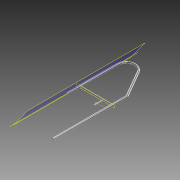
# Autodesk Inventor part: Geländer lang
Saved by Autodesk Inventor 2019 (Build 230136000, 136)
## iProperties
Created: 2017-04-11
Part Number: Geländer lang
Material: Allgemein
Document SubType Name: Modeling
Designer: Seelenernter
Density: 1 g/cm^3
Appearance: Chrom - poliert
Author: Seelenernter
Autodesk Inventor part; units mm, degrees
ref_plane "YZ Plane" through (0, 0, 0) normal (1, 0, 0) x (0, 1, 0)
ref_plane "XY Plane" through (0, 0, 0) normal (0, 0, 1) x (1, 0, 0)
sketch "Skizze1" plane through (0, 0, 0) normal (0, 1, 0) x (-1, 0, 0)
  circle A0 centre (0, 0) radius 20
  dimension "d0" = 40
  constraints: 1 centre point, 1 coincident
  measures "d0" diameter of A0
sketch "Skizze2" plane through (0, 0, 0) normal (0, 0, 1) x (1, 0, 0)
  line L0 (0, 0) -> (0, 770)
  line L1 (180, 950) -> (183.4788, 950)
  line L2 (356.6838, 850) -> (680, 290)
  line L3 (680, 290) -> (680, -1250)
  arc A0 (180, 950) -> (0, 770) centre (180, 770) ccw
  arc A1 (356.6838, 850) -> (183.4788, 950) centre (183.4788, 750) ccw
  point P0 (0, 950)
  dimension "d1" = 950
  dimension "d4" = 290
  dimension "d8" = 2200
  dimension "d9" = 30
  dimension "d10" = 680
  dimension "d11" = 180
  dimension "d12" = 200
  constraints: 8 end point, 4 point on circle, 4 tangent, 2 centre point, 2 point on line, 2 vertical, 1 perpendicular
  measures "d1" distance of L0.start point (0, 950)
  measures "d4" vertical distance of L2.end L0.start
  measures "d8" distance from line of L3.end L1
  measures "d9" angle of L2 L3
  measures "d10" distance between parallel lines of L0 L3
  measures "d11" radius of A0
  measures "d12" radius of A1
sweep "Sweeping1" add profiles "Skizze1" path "Skizze2"
sketch "Skizze3" plane through (0, 0, 0) normal (1, 0, 0) x (0, 1, 0)
  circle A0 centre (-20, 0) radius 15
  line L0 (0, 20) -> (0, -20) projected
  point P0 (0, 0)
  point P1 (0, 0)
  dimension "d16" = 30
  dimension "d27" = 20
  constraints: 1 centre point, 1 horizontal alignment, 1 midpoint
  measures "d16" diameter of A0
  measures "d27" distance from line of L0 A0.centre
extrude "Extrusion1" add sketch "Skizze3" along normal blind 680
sketch "Skizze4" plane through (0, 0, 0) normal (0, -1, 0) x (1, 0, 0)
  circle A0 centre (0, 0) radius 20 projected
extrude "Extrusion2" add sketch "Skizze4" along normal blind 100
ref_plane "Arbeitsebene1" through (0, -20, 0) normal (0, 1, 0) x (-1, 0, 0)
sketch "Skizze5" plane through (0, -20, 0) normal (0, 1, 0) x (-1, 0, 0)
  circle A0 centre (0, 0) radius 20 projected
  circle A1 centre (-500, 0) radius 15
  dimension "d23" = 30
  dimension "d24" = 500
  constraints: 1 centre point
  measures "d23" diameter of A1
  measures "d24" distance of point (0, 0) A1.centre
extrude "Extrusion3" add sketch "Skizze5" against normal blind 200 contours A1
ref_plane "Arbeitsebene2" through (500, -160, 0) normal (0, -1, 0) x (1, 0, 0)
sketch "Skizze6" plane through (500, -160, 0) normal (0, -1, 0) x (1, 0, 0)
  circle A0 centre (0, 0) radius 15 projected
  circle A1 centre (180, 0) radius 20 projected
  circle A2 centre (180, 0) radius 20 projected
  circle A3 centre (0, 0) radius 15 projected
  line L0 (0, 15) -> (180, 15)
  line L1 (180, 15) -> (180, -15)
  line L2 (180, -15) -> (0, -15)
  line L3 (0, -15) -> (0, 15)
  point P0 (-500, 0)
  dimension "d29" = 0
  dimension "d30" = 0
  dimension "d31" = 30
  dimension "d32" = 15
  constraints: 8 end point, 2 parallel, 1 horizontal, 1 perpendicular
  measures "d29" distance from line of A1.centre L1
  measures "d30" distance from line of A0.centre L3
  measures "d31" distance of L2.end L0.start
  measures "d32" distance from line of A0.centre L2
extrude "Extrusion4" add sketch "Skizze6" along normal blind 5 contours A0 L3 | A0 L0 A1 L2 | L0 L1 L2 A1 picked at (3.1174, 3.9092) picked at (173.3822, 0.8057)
sketch "Skizze7" plane through (0, -100, 0) normal (0, -1, 0) x (1, 0, 0)
  circle A0 centre (0, 0) radius 20 projected
  circle A1 centre (0, 0) radius 15
  dimension "d35" = 30
  constraints: 1 centre point, 1 coincident
  measures "d35" diameter of A1
extrude "Extrusion5" add sketch "Skizze7" along normal blind 190 contours A1
ref_plane "Arbeitsebene3" through (0, -100, 0) normal (-0.8086, 0, 0.5883) x (0, -1, 0)
sketch "Skizze8" plane through (0, -100, 0) normal (-0.8086, 0, 0.5883) x (0, -1, 0)
  line L0 (190, -15) -> (190, 15) projected
  line L1 (0, 15) -> (0, -15) projected
  point P0 (-100, 0)
  point P1 (177.8177, 0)
hole "Bohrung1" at (0, -277.8177, 0) direction (0.8086, 0, -0.5883) diameter 5 end through all both
